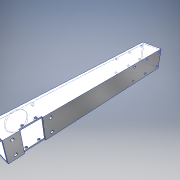
# Autodesk Inventor part: Arm 18 inch
Saved by Autodesk Inventor 2019 (Build 230136000, 136)
## iProperties
Created: 2018-09-22
Part Number: Arm 18 inch
Material: Aluminum 6061
Document SubType Name: Modeling
Designer: Adhik
Density: 2.7 g/cm^3
Appearance: Aluminum - Flat
Mass: 627.711 g
Surface Area: 1498.7 cm^2
Volume: 232.486 cm^3
Author: Adhik
Autodesk Inventor part; units mm, degrees
ref_plane "YZ Plane" through (0, 0, 0) normal (1, 0, 0) x (0, 1, 0)
ref_plane "XZ Plane" through (0, 0, 0) normal (0, 1, 0) x (-1, 0, 0)
ref_plane "XY Plane" through (0, 0, 0) normal (0, 0, 1) x (1, 0, 0)
sketch "Sketch1" plane through (0, 0, 0) normal (0, 0, 1) x (1, 0, 0)
  line L0 (-35.56, 0) -> (35.56, 0) construction
  line L1 (0, -35.56) -> (0, 35.56) construction
  line L2 (-25.4, 25.4) -> (25.4, 25.4)
  line L3 (25.4, 25.4) -> (25.4, -25.4)
  line L4 (25.4, -25.4) -> (-25.4, -25.4)
  line L5 (-25.4, -25.4) -> (-25.4, 25.4)
  line L6 (-22.225, 22.225) -> (22.225, 22.225)
  line L7 (22.225, 22.225) -> (22.225, -22.225)
  line L8 (22.225, -22.225) -> (-22.225, -22.225)
  line L9 (-22.225, -22.225) -> (-22.225, 22.225)
  point P0 (0, 0)
  point P1 (-25.4, 0)
  point P2 (0, 25.4)
  point P3 (-22.225, 0)
  point P4 (0, 22.225)
  dimension "d0" = 50.8
  dimension "d1" = 3.175
  constraints: 16 end point, 4 midpoint, 4 parallel, 4 perpendicular, 4 point on line, 2 horizontal
  measures "d0" distance of L4.end L2.start
  measures "d1" distance between parallel lines of L2 L6
extrude "Extrusion1" add sketch "Sketch1" along normal mid plane 406.4
sketch "Sketch2" plane through (25.4, -25.4, 203.2) normal (1, 0, 0) x (0, 0, -1)
  line L0 (542.6964, 25.4) -> (-90.4494, 25.4) construction
  line L1 (203.2, -10.16) -> (203.2, 60.96) construction
  line L2 (309.88, 7.62) -> (398.78, 7.62) construction
  line L3 (398.78, 7.62) -> (398.78, 43.18) construction
  line L4 (398.78, 43.18) -> (309.88, 43.18) construction
  line L5 (309.88, 43.18) -> (309.88, 7.62) construction
  circle A0 centre (309.88, 43.18) radius 2.667
  circle A1 centre (309.88, 7.62) radius 2.667
  circle A2 centre (354.33, 7.62) radius 2.667
  circle A3 centre (398.78, 7.62) radius 2.667
  circle A4 centre (398.78, 43.18) radius 2.667
  circle A5 centre (354.33, 43.18) radius 2.667
  line L6 (406.4, 50.8) -> (406.4, 0) construction
  point P0 (203.2, 25.4)
  point P1 (398.78, 25.4)
  dimension "d4" = 5.334
  dimension "d5" = 7.62
  dimension "d6" = 88.9
  dimension "d7" = 17.78
  constraints: 8 end point, 6 centre point, 5 equal radius, 4 coincident, 3 midpoint, 2 parallel, 1 horizontal, 1 perpendicular, 1 point on line
  measures "d4" diameter of A1
  measures "d5" distance between parallel lines of L6 L3
  measures "d6" distance of L3.end L4.end
  measures "d7" distance between parallel lines of L0 L4
extrude "Extrusion2" cut sketch "Sketch2" against normal through all
sketch "Sketch10" plane through (25.4, -25.4, 203.2) normal (1, 0, 0) x (0, 0, -1)
  line L0 (487.68, 25.4) -> (-81.28, 25.4) construction
  circle A0 centre (398.78, 43.18) radius 2.667 construction
  circle A1 centre (354.33, 7.62) radius 2.667 construction
  circle A2 centre (309.88, 43.18) radius 2.667 construction
  circle A3 centre (309.88, 7.62) radius 2.667 construction
  circle A4 centre (398.78, 7.62) radius 2.667 construction
  circle A5 centre (354.33, 43.18) radius 2.667 construction
  line L1 (0, 50.8) -> (406.4, 50.8) construction
  line L2 (0, 0) -> (0, 50.8) construction
  line L3 (0, 0) -> (406.4, 0) construction
  line L4 (406.4, 50.8) -> (406.4, 0) construction
  line L5 (29.7942, 50.8) -> (71.8058, 50.8)
  line L6 (71.8058, 50.8) -> (71.8058, 0)
  line L7 (71.8058, 0) -> (29.7942, 0)
  line L8 (29.7942, 0) -> (29.7942, 50.8)
  line L9 (29.7942, 50.8) -> (71.8058, 0) construction
  point P0 (203.2, 25.4)
  point P1 (50.8, 25.4)
  point P2 (29.7942, 25.4)
  dimension "d47" = 50.8
  dimension "d48" = 42.0116
  dimension "d49" = 50.8
  constraints: 10 end point, 2 midpoint, 2 parallel, 1 horizontal, 1 perpendicular, 1 point on line
  measures "d47" distance of L7.end L5.start
  measures "d48" distance of L5.start L5.end
  measures "d49" distance from line of L2 point (50.8, 25.4)
extrude "Extrusion9" cut sketch "Sketch10" against normal blind 3.175
sketch "Sketch11" plane through (-25.4, 25.4, -203.2) normal (0, 1, 0) x (1, 0, 0)
  circle A0 centre (43.7, -368.3) radius 2.0193 construction
  circle A1 centre (43.7, -342.9) radius 2.0193 construction
  circle A2 centre (43.7, -342.9) radius 2.413
  circle A3 centre (43.7, -368.3) radius 2.413
  point P0 (25.4, -203.2)
  dimension "d73" = 4.826
  constraints: 4 centre point, 2 coincident, 1 equal radius, 4 other
  measures "d73" diameter of A2
sketch "Sketch12" plane through (-25.4, -25.4, 203.2) normal (-1, 0, 0) x (0, 0, 1)
  line L0 (-487.68, 25.4) -> (81.28, 25.4) construction
  circle A0 centre (-398.78, 43.18) radius 2.667 construction
  circle A1 centre (-354.33, 7.62) radius 2.667 construction
  circle A2 centre (-309.88, 43.18) radius 2.667 construction
  circle A3 centre (-309.88, 7.62) radius 2.667 construction
  circle A4 centre (-398.78, 7.62) radius 2.667 construction
  circle A5 centre (-354.33, 43.18) radius 2.667 construction
  line L1 (0, 0) -> (-406.4, 0) construction
  line L2 (0, 50.8) -> (0, 0) construction
  line L3 (-406.4, 50.8) -> (0, 50.8) construction
  line L4 (-406.4, 0) -> (-406.4, 50.8) construction
  circle A6 centre (-50.8, 25.4) radius 22.225
  point P0 (-203.2, 25.4)
  dimension "d54" = 50.8
  dimension "d55" = 44.45
  constraints: 1 centre point, 1 point on line
  measures "d54" distance from line of L2 A6.centre
  measures "d55" diameter of A6
extrude "Extrusion11" cut sketch "Sketch12" against normal blind 3.175
sketch "Sketch14" plane through (22.225, -22.225, -203.2) normal (-1, 0, 0) x (0, 0, 1)
  line L0 (-81.28, 22.225) -> (487.68, 22.225) construction
  circle A0 centre (355.6, 22.225) radius 22.225 construction
  line L1 (355.6, 0) -> (355.6, 44.45) construction
  line L2 (391.5029, 6.35) -> (319.6971, 6.35) construction
  line L3 (319.6971, 6.35) -> (319.6971, 38.1) construction
  line L4 (319.6971, 38.1) -> (391.5029, 38.1) construction
  line L5 (391.5029, 38.1) -> (391.5029, 6.35) construction
  circle A1 centre (391.5029, 6.35) radius 3.175
  circle A2 centre (391.5029, 38.1) radius 3.175
  circle A3 centre (319.6971, 6.35) radius 3.175
  circle A4 centre (319.6971, 38.1) radius 3.175
  line L6 (406.4, 0) -> (376.6058, 0) projected
  point P0 (203.2, 22.225)
  point P1 (391.5029, 22.225)
  point P2 (391.5029, 0)
  dimension "d67" = 6.35
  dimension "d68" = 31.75
  constraints: 10 end point, 5 coincident, 4 centre point, 3 equal radius, 3 midpoint, 2 parallel, 2 perpendicular, 2 point on line, 1 horizontal, 1 vertical alignment, 2 other
  measures "d67" diameter of A3
  measures "d68" distance of L4.end L2.start
extrude "Extrusion12" cut sketch "Sketch14" against normal through all
sketch "Sketch15" plane through (-25.4, -25.4, 203.2) normal (-1, 0, 0) x (0, 0, 1)
  circle A0 centre (-86.7029, 9.525) radius 3.175 projected
  circle A1 centre (-86.7029, 41.275) radius 3.175 projected
  point P0 (-203.2, 25.4)
extrude "Extrusion13" cut sketch "Sketch15" against normal up to next
extrude "Extrusion14" cut sketch "Sketch11" against normal through all
body "Solid1"
